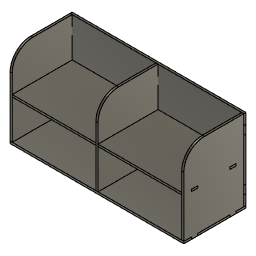
cad v1 (Autodesk Fusion 360 design; units mm, degrees)
Autodesk Fusion 360 part; units mm, degrees
sketch "Sketch1" plane through (0, 0, 0) normal (0, 0, 1) x (1, 0, 0)
  line L0 (-210, 150) -> (210, 150)
  line L1 (210, 150) -> (210, 0)
  line L2 (210, 0) -> (-210, 0)
  line L3 (-210, 0) -> (-210, 150)
  dimension "d6" = 420
  dimension "d7" = 150
  constraint horizontal L0
  constraint vertical L1
  constraint horizontal L2
  constraint vertical L3
  constraint coincident origin L2
  constraint midpoint L2 origin
  measures "d6" distance of L0.start L0.end
  measures "d7" distance of L0.start L2.end
extrude "Extrude1" add sketch "Sketch1" along normal blind 5 makes body 1
sketch "Sketch4" plane through (0, 150, 0) normal (0, 1, 0) x (-1, 0, 0)
  line L0 (-210, 0) -> (210, 0)
  line L1 (210, 0) -> (210, 5)
  line L2 (210, 5) -> (-210, 5)
  line L3 (-210, 5) -> (-210, 0)
  line L4 (-210, 5) -> (210, 5)
  line L5 (210, 5) -> (210, 200)
  line L6 (210, 200) -> (-210, 200)
  line L7 (-210, 200) -> (-210, 5)
  line L8 (115.5, 0) -> (157.5, 0)
  line L9 (157.5, 0) -> (157.5, 5)
  line L10 (157.5, 5) -> (115.5, 5)
  line L11 (115.5, 5) -> (115.5, 0)
  line L12 (-157.5, 0) -> (-115.5, 0)
  line L13 (-115.5, 0) -> (-115.5, 5)
  line L14 (-115.5, 5) -> (-157.5, 5)
  line L15 (-157.5, 5) -> (-157.5, 0)
  line L16 (-21, 5) -> (21, 5)
  line L17 (21, 5) -> (21, 0)
  line L18 (21, 0) -> (-21, 0)
  line L19 (-21, 0) -> (-21, 5)
  point P0 (0, 5)
  point P1 (0, 5)
  point P2 (0, 5)
  dimension "d10" = 420
  dimension "d11" = 195
  dimension "d39" = 42
  dimension "d40" = 5
  dimension "d41" = 52.5
  dimension "d42" = 42
  dimension "d43" = 5
  dimension "d44" = 52.5
  dimension "d45" = 42
  dimension "d46" = 5
  constraint horizontal L4
  constraint vertical L5
  constraint horizontal L6
  constraint vertical L7
  constraint midpoint L2 P2
  constraint midpoint L4 P2
  constraint coincident P2 P1
  constraint horizontal L8
  constraint vertical L9
  constraint horizontal L10
  constraint vertical L11
  constraint horizontal L12
  constraint vertical L13
  constraint horizontal L14
  constraint vertical L15
  constraint coincident L4 L10.end
  constraint coincident L4 L13.end
  constraint horizontal L16
  constraint vertical L17
  constraint horizontal L18
  constraint vertical L19
  constraint midpoint L16 P2
  measures "d10" distance of L2.end L1.end
  measures "d11" distance of L2.end L6.end
  measures "d39" distance of L8.start L8.end
  measures "d40" distance of L8.end L9.end
  measures "d41" horizontal distance of L1.end L8.end
  measures "d42" distance of L12.start L12.end
  measures "d43" distance of L12.start L14.end
  measures "d44" horizontal distance of L2.end L14.end
  measures "d45" distance of L17.end L18.end
  measures "d46" distance of L16.start L18.end
extrude "Extrude2" add sketch "Sketch4" against normal blind 5 separate body contours L0 L2 L4 L12 L13 L14 L15 | L2 L4 L5 L6 L7 L10 L14 L16 | L0 L2 L4 L16 L17 L18 L19 | L0 L2 L4 L8 L9 L10 L11 makes body 2
sketch "Sketch5" plane through (210, 0, 0) normal (1, 0, 0) x (0, 1, 0)
  line L0 (0, 0) -> (150, 0)
  line L1 (150, 0) -> (150, 5)
  line L2 (150, 5) -> (0, 5)
  line L3 (0, 5) -> (0, 0)
  line L4 (0, 5) -> (145, 5)
  line L5 (145, 5) -> (145, 200)
  line L6 (145, 200) -> (0, 200)
  line L7 (0, 200) -> (0, 5)
  line L8 (18.75, 5) -> (33.75, 5)
  line L9 (33.75, 5) -> (33.75, 0)
  line L10 (33.75, 0) -> (18.75, 0)
  line L11 (18.75, 0) -> (18.75, 5)
  line L12 (111.25, 5) -> (126.25, 5)
  line L13 (126.25, 5) -> (126.25, 0)
  line L14 (126.25, 0) -> (111.25, 0)
  line L15 (111.25, 0) -> (111.25, 5)
  line L16 (145, 30) -> (150, 30)
  line L17 (150, 30) -> (150, 50)
  line L18 (150, 50) -> (145, 50)
  line L19 (145, 50) -> (145, 30)
  line L20 (145, 155) -> (150, 155)
  line L21 (150, 155) -> (150, 175)
  line L22 (150, 175) -> (145, 175)
  line L23 (145, 175) -> (145, 155)
  point P0 (145, 5)
  dimension "d14" = 145
  dimension "d15" = 195
  dimension "d27" = 20
  dimension "d28" = 5
  dimension "d29" = 25
  dimension "d30" = 20
  dimension "d31" = 5
  dimension "d32" = 25
  dimension "d33" = 15
  dimension "d34" = 5
  dimension "d35" = 18.75
  dimension "d36" = 15
  dimension "d37" = 5
  dimension "d38" = 18.75
  constraint horizontal L4
  constraint vertical L5
  constraint horizontal L6
  constraint vertical L7
  constraint coincident P0 L4.end
  constraint horizontal L8
  constraint vertical L9
  constraint horizontal L10
  constraint vertical L11
  constraint horizontal L12
  constraint vertical L13
  constraint horizontal L14
  constraint vertical L15
  constraint horizontal L16
  constraint vertical L17
  constraint horizontal L18
  constraint vertical L19
  constraint horizontal L20
  constraint vertical L21
  constraint horizontal L22
  constraint vertical L23
  constraint coincident L5 L18.end
  constraint coincident L5 L22.end
  constraint coincident L4 L12.start
  constraint coincident L4 L8.end
  measures "d14" distance of L2.end P0
  measures "d15" distance of L2.end L6.end
  measures "d27" distance of L16.end L17.end
  measures "d28" distance of L16.start L16.end
  measures "d29" vertical distance of P0 L16.end
  measures "d30" distance of L20.end L21.end
  measures "d31" distance of L20.start L20.end
  measures "d32" vertical distance of L5.end L21.end
  measures "d33" distance of L13.end L14.end
  measures "d34" distance of L12.end L13.end
  measures "d35" horizontal distance of P0 L13.end
  measures "d36" distance of L9.end L10.end
  measures "d37" distance of L8.end L9.end
  measures "d38" horizontal distance of L2.end L10.end
extrude "Extrude3" add sketch "Sketch5" against normal blind 5 separate body contours L0 L2 L4 L8 L9 L10 L11 | L2 L4 L5 L6 L7 L8 L12 L19 L23 | L0 L2 L4 L12 L13 L14 L15 | L5 L20 L21 L22 L23 | L5 L16 L17 L18 L19 makes body 3
fillet "Fillet1" radius 50 1 edges at (207.5, 0, 200) on bodies 3
pattern_linear "R-Pattern1" count 3 spacing 207.5 along (-1, 0, 0) of bodies 3 makes body 4 at (2.5, 59.5833, 68.3333) makes body 5 at (-205, 59.5833, 68.3333)
ref_plane "WorkPlane1" through (0, 75, 100) normal (0, 0, -1) x (-1, 0, 0)
sketch "Sketch6" plane through (0, 0, 100) normal (0, 0, -1) x (-1, 0, 0)
  line L0 (205, 145) -> (-205, 145)
  line L1 (-205, 145) -> (-205, 0)
  line L2 (-205, 0) -> (205, 0)
  line L3 (205, 0) -> (205, 145)
  line L4 (210, 126.25) -> (205, 126.25)
  line L5 (205, 126.25) -> (205, 111.25)
  line L6 (205, 111.25) -> (210, 111.25)
  line L7 (210, 111.25) -> (210, 126.25)
  line L8 (210, 33.75) -> (205, 33.75)
  line L9 (205, 33.75) -> (205, 18.75)
  line L10 (205, 18.75) -> (210, 18.75)
  line L11 (210, 18.75) -> (210, 33.75)
  line L12 (152.5, 150) -> (110.5, 150)
  line L13 (110.5, 150) -> (110.5, 145)
  line L14 (110.5, 145) -> (152.5, 145)
  line L15 (152.5, 145) -> (152.5, 150)
  line L16 (21, 150) -> (-21, 150)
  line L17 (-21, 150) -> (-21, 145)
  line L18 (-21, 145) -> (21, 145)
  line L19 (21, 145) -> (21, 150)
  line L20 (2.5, 75) -> (-2.5, 75)
  line L21 (-2.5, 75) -> (-2.5, 0)
  line L22 (-2.5, 0) -> (2.5, 0)
  line L23 (2.5, 0) -> (2.5, 75)
  line L24 (0, 1.75) -> (0, 22.5)
  line L25 (-110.5, 145) -> (-152.5, 145)
  line L26 (-152.5, 145) -> (-152.5, 150)
  line L27 (-152.5, 150) -> (-110.5, 150)
  line L28 (-110.5, 150) -> (-110.5, 145)
  line L29 (-205, 126.25) -> (-205, 111.25)
  line L30 (-205, 111.25) -> (-210, 111.25)
  line L31 (-210, 126.25) -> (-205, 126.25)
  line L32 (-210, 111.25) -> (-210, 126.25)
  line L33 (-205, 33.75) -> (-205, 18.75)
  line L34 (-205, 18.75) -> (-210, 18.75)
  line L35 (-210, 33.75) -> (-205, 33.75)
  line L36 (-210, 18.75) -> (-210, 33.75)
  point P0 (205, 145)
  point P1 (-205, 0)
  point P2 (0, 145)
  point P3 (0, 145)
  dimension "d47" = 75
  dimension "d48" = 5
  dimension "d49" = 15
  dimension "d50" = 5
  dimension "d51" = 18.75
  dimension "d52" = 15
  dimension "d53" = 5
  dimension "d54" = 18.75
  dimension "d55" = 42
  dimension "d56" = 5
  dimension "d57" = 52.5
  dimension "d58" = 42
  dimension "d59" = 5
  constraint horizontal L0
  constraint vertical L1
  constraint horizontal L2
  constraint vertical L3
  constraint coincident P0 L0.start
  constraint coincident P1 L1.end
  constraint horizontal L4
  constraint vertical L5
  constraint horizontal L6
  constraint vertical L7
  constraint horizontal L8
  constraint vertical L9
  constraint horizontal L10
  constraint vertical L11
  constraint horizontal L12
  constraint vertical L13
  constraint horizontal L14
  constraint vertical L15
  constraint horizontal L16
  constraint vertical L17
  constraint horizontal L18
  constraint vertical L19
  constraint horizontal L20
  constraint vertical L21
  constraint horizontal L22
  constraint vertical L23
  constraint midpoint L22 origin
  constraint coincident L3 L5.end
  constraint coincident L3 L8.end
  constraint coincident L0 L13.end
  constraint midpoint L18 P3
  constraint midpoint L0 P3
  constraint coincident P3 P2
  constraint symmetric L4.start L24 L31.start
  constraint symmetric L4.end L24 L29.start
  constraint symmetric L5.end L24 L29.end
  constraint symmetric L6.end L24 L30.end
  constraint symmetric L8.start L24 L35.start
  constraint symmetric L8.end L24 L33.start
  constraint symmetric L9.end L24 L33.end
  constraint symmetric L10.end L24 L34.end
  constraint symmetric L12.start L24 L26.end
  constraint symmetric L12.end L24 L27.end
  constraint symmetric L13.end L24 L25.start
  constraint symmetric L14.end L24 L25.end
  measures "d47" distance of L20.end L21.end
  measures "d48" distance of L20.start L20.end
  measures "d49" distance of L4.start L6.end
  measures "d50" distance of L4.start L4.end
  measures "d51" vertical distance of P0 L4.start
  measures "d52" distance of L8.start L10.end
  measures "d53" distance of L9.end L10.end
  measures "d54" vertical distance of L2.end L10.end
  measures "d55" distance of L12.start L12.end
  measures "d56" distance of L12.start L14.end
  measures "d57" horizontal distance of P0 L12.start
  measures "d58" distance of L16.start L16.end
  measures "d59" distance of L16.start L18.end
extrude "Extrude4" add sketch "Sketch6" against normal blind 5 separate body contours L0 L1 L2 L3 L5 L9 L14 L18 L20 L21 L23 L25 L29 L33 | L0 L12 L13 L14 L15 | L3 L4 L5 L6 L7 | L0 L16 L17 L18 L19 | L3 L8 L9 L10 L11 | L0 L25 L26 L27 L28 | L1 L29 L30 L31 L32 | L1 L33 L34 L35 L36 makes body 6
combine "Combine1" operation cut target body 1 tool bodies 3 5 2 4 keep tools
combine "Combine2" operation cut target body 4 tool bodies 6 keep tools
combine "Combine3" operation cut target body 3 tool bodies 6 keep tools
combine "Combine4" operation cut target body 2 tool bodies 6 keep tools
combine "Combine5" operation cut target body 5 tool bodies 6 keep tools
equation "len = 420 mm"
equation "dep = 150 mm"
equation "hei = 200 mm"
equation "t = 5 mm"
equation "fil = 50 mm"
equation "d6 = len"
equation "d7 = dep"
equation "d8 = t"
equation "d10 = len"
equation "d11 = hei - t"
equation "d12 = -t"
equation "d14 = dep - t"
equation "d15 = hei - t"
equation "d16 = -t"
equation "d19 = fil"
equation "d22 = len - t"
equation "d24 = -( hei / 2 )"
equation "d25 = -t"
equation "d27 = hei / 10"
equation "d28 = t"
equation "d29 = hei / 8"
equation "d30 = d27"
equation "d31 = d28"
equation "d32 = d29"
equation "d33 = dep / 10"
equation "d34 = t"
equation "d35 = dep / 8"
equation "d36 = d33"
equation "d37 = d34"
equation "d38 = d35"
equation "d39 = len / 10"
equation "d40 = t"
equation "d41 = len / 8"
equation "d42 = d39"
equation "d43 = d40"
equation "d44 = d41"
equation "d45 = d39"
equation "d46 = d43"
equation "d47 = dep / 2"
equation "d48 = t"
equation "d49 = dep / 10"
equation "d50 = t"
equation "d51 = dep / 8"
equation "d52 = d49"
equation "d53 = d50"
equation "d54 = d51"
equation "d55 = len / 10"
equation "d56 = t"
equation "d57 = len / 8"
equation "d58 = len / 10"
equation "d59 = t"
